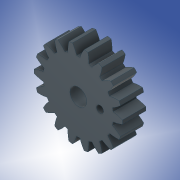
# Autodesk Inventor part: GA002
Saved by Autodesk Inventor 2017 SP1 (Build 210196100, 196)
## iProperties
Created: 2017-06-20
Part Number: GA002
Material: ABS Plastic
Document SubType Name: Modeling
Designer: zallen
Density: 1.06 g/cm^3
Appearance: CR Dark Blue
Author: zallen
Autodesk Inventor part; units mm, degrees
ref_plane "YZ Plane" through (0, 0, 0) normal (1, 0, 0) x (0, 1, 0)
ref_plane "XZ Plane" through (0, 0, 0) normal (0, 1, 0) x (-1, 0, 0)
ref_plane "XY Plane" through (0, 0, 0) normal (0, 0, 1) x (1, 0, 0)
sketch "Sketch1" plane through (0, 0, 0) normal (0, 0, 1) x (1, 0, 0)
  circle A0 centre (0, 0) radius 15
  circle A1 centre (0, 0) radius 3.6
  dimension "d0" = 30
  dimension "d1" = 7.2
  constraints: 2 centre point, 2 coincident
  measures "d0" diameter of A0
  measures "d1" diameter of A1
extrude "Extrusion1" add sketch "Sketch1" along normal blind 10
sketch "Sketch2" plane through (0, 0, 10) normal (0, 0, 1) x (1, 0, 0)
  circle A0 centre (9.3, 0) radius 1.5
  circle A1 centre (0, 0) radius 15 construction
  circle A2 centre (0, 0) radius 3.6 construction
  line L0 (3.6, 0) -> (15, 0) construction
  circle A3 centre (0, 0) radius 3.6 construction
  circle A4 centre (0, 0) radius 15 construction
  dimension "d4" = 3
  constraints: 5 horizontal alignment, 2 coincident, 2 end point, 1 centre point, 1 horizontal, 1 midpoint, 4 other
  measures "d4" diameter of A0
extrude "Extrusion2" cut sketch "Sketch2" against normal through all
sketch "Sketch3" plane through (0, 0, 10) normal (0, 0, 1) x (1, 0, 0)
  line L0 (0, 0) -> (25, 0) construction
  arc A0 (18.8792, 0.8) -> (14.8792, 1.9) centre (12.94, -12.9741) ccw
  circle A1 centre (0, 0) radius 15 projected
  arc A2 (18.8792, -0.8) -> (18.8792, 0.8) centre (-1.1048, 0) ccw
  arc A3 (14.8792, -1.9) -> (18.8792, -0.8) centre (12.94, 12.9741) ccw
  arc A4 (14.8792, -1.9) -> (14.8792, 1.9) centre (0, 0) ccw
  arc A5 (17.467, 7.2088) -> (13.332, 6.8744) centre (16.5971, -7.7659) ccw
  arc A6 (18.0142, 5.7053) -> (17.467, 7.2088) centre (-1.0382, -0.3779) ccw
  arc A7 (14.6317, 3.3036) -> (18.0142, 5.7053) centre (7.7223, 16.6175) ccw
  arc A8 (14.6317, 3.3036) -> (13.332, 6.8744) centre (0, 0) ccw
  arc A9 (13.9481, 12.7481) -> (10.1768, 11.0196) centre (18.2523, -1.6211) ccw
  arc A10 (14.9765, 11.5225) -> (13.9481, 12.7481) centre (-0.8463, -0.7102) ccw
  arc A11 (12.6194, 8.1087) -> (14.9765, 11.5225) centre (1.573, 18.2565) ccw
  arc A12 (12.6194, 8.1087) -> (10.1768, 11.0196) centre (0, 0) ccw
  arc A13 (8.7468, 16.7498) -> (5.7941, 13.8357) centre (17.7059, 4.7193) ccw
  arc A14 (10.1324, 15.9498) -> (8.7468, 16.7498) centre (-0.5524, -0.9568) ccw
  arc A15 (9.085, 11.9357) -> (10.1324, 15.9498) centre (-4.7659, 17.6935) ccw
  arc A16 (9.085, 11.9357) -> (5.7941, 13.8357) centre (0, 0) ccw
  arc A17 (2.4905, 18.7313) -> (0.7126, 14.9831) centre (15.024, 10.4905) ccw
  arc A18 (4.0662, 18.4534) -> (2.4905, 18.7313) centre (-0.1918, -1.088) ccw
  arc A19 (4.4549, 14.3232) -> (4.0662, 18.4534) centre (-10.53, 14.9964) ccw
  arc A20 (4.4549, 14.3232) -> (0.7126, 14.9831) centre (0, 0) ccw
  arc A21 (-4.0662, 18.4534) -> (-4.4549, 14.3232) centre (10.53, 14.9964) ccw
  arc A22 (-2.4905, 18.7313) -> (-4.0662, 18.4534) centre (0.1918, -1.088) ccw
  arc A23 (-0.7126, 14.9831) -> (-2.4905, 18.7313) centre (-15.024, 10.4905) ccw
  arc A24 (-0.7126, 14.9831) -> (-4.4549, 14.3232) centre (0, 0) ccw
  arc A25 (-10.1324, 15.9498) -> (-9.085, 11.9357) centre (4.7659, 17.6935) ccw
  arc A26 (-8.7468, 16.7498) -> (-10.1324, 15.9498) centre (0.5524, -0.9568) ccw
  arc A27 (-5.7941, 13.8357) -> (-8.7468, 16.7498) centre (-17.7059, 4.7193) ccw
  arc A28 (-5.7941, 13.8357) -> (-9.085, 11.9357) centre (0, 0) ccw
  arc A29 (-14.9765, 11.5225) -> (-12.6194, 8.1087) centre (-1.573, 18.2565) ccw
  arc A30 (-13.9481, 12.7481) -> (-14.9765, 11.5225) centre (0.8463, -0.7102) ccw
  arc A31 (-10.1768, 11.0196) -> (-13.9481, 12.7481) centre (-18.2523, -1.6211) ccw
  arc A32 (-10.1768, 11.0196) -> (-12.6194, 8.1087) centre (0, 0) ccw
  arc A33 (-18.0142, 5.7053) -> (-14.6317, 3.3036) centre (-7.7223, 16.6175) ccw
  arc A34 (-17.467, 7.2088) -> (-18.0142, 5.7053) centre (1.0382, -0.3779) ccw
  arc A35 (-13.332, 6.8744) -> (-17.467, 7.2088) centre (-16.5971, -7.7659) ccw
  arc A36 (-13.332, 6.8744) -> (-14.6317, 3.3036) centre (0, 0) ccw
  arc A37 (-18.8792, -0.8) -> (-14.8792, -1.9) centre (-12.94, 12.9741) ccw
  arc A38 (-18.8792, 0.8) -> (-18.8792, -0.8) centre (1.1048, 0) ccw
  arc A39 (-14.8792, 1.9) -> (-18.8792, 0.8) centre (-12.94, -12.9741) ccw
  arc A40 (-14.8792, 1.9) -> (-14.8792, -1.9) centre (0, 0) ccw
  arc A41 (-17.467, -7.2088) -> (-13.332, -6.8744) centre (-16.5971, 7.7659) ccw
  arc A42 (-18.0142, -5.7053) -> (-17.467, -7.2088) centre (1.0382, 0.3779) ccw
  arc A43 (-14.6317, -3.3036) -> (-18.0142, -5.7053) centre (-7.7223, -16.6175) ccw
  arc A44 (-14.6317, -3.3036) -> (-13.332, -6.8744) centre (0, 0) ccw
  arc A45 (-13.9481, -12.7481) -> (-10.1768, -11.0196) centre (-18.2523, 1.6211) ccw
  arc A46 (-14.9765, -11.5225) -> (-13.9481, -12.7481) centre (0.8463, 0.7102) ccw
  arc A47 (-12.6194, -8.1087) -> (-14.9765, -11.5225) centre (-1.573, -18.2565) ccw
  arc A48 (-12.6194, -8.1087) -> (-10.1768, -11.0196) centre (0, 0) ccw
  arc A49 (-8.7468, -16.7498) -> (-5.7941, -13.8357) centre (-17.7059, -4.7193) ccw
  arc A50 (-10.1324, -15.9498) -> (-8.7468, -16.7498) centre (0.5524, 0.9568) ccw
  arc A51 (-9.085, -11.9357) -> (-10.1324, -15.9498) centre (4.7659, -17.6935) ccw
  arc A52 (-9.085, -11.9357) -> (-5.7941, -13.8357) centre (0, 0) ccw
  arc A53 (-2.4905, -18.7313) -> (-0.7126, -14.9831) centre (-15.024, -10.4905) ccw
  arc A54 (-4.0662, -18.4534) -> (-2.4905, -18.7313) centre (0.1918, 1.088) ccw
  arc A55 (-4.4549, -14.3232) -> (-4.0662, -18.4534) centre (10.53, -14.9964) ccw
  arc A56 (-4.4549, -14.3232) -> (-0.7126, -14.9831) centre (0, 0) ccw
  arc A57 (4.0662, -18.4534) -> (4.4549, -14.3232) centre (-10.53, -14.9964) ccw
  arc A58 (2.4905, -18.7313) -> (4.0662, -18.4534) centre (-0.1918, 1.088) ccw
  arc A59 (0.7126, -14.9831) -> (2.4905, -18.7313) centre (15.024, -10.4905) ccw
  arc A60 (0.7126, -14.9831) -> (4.4549, -14.3232) centre (0, 0) ccw
  arc A61 (10.1324, -15.9498) -> (9.085, -11.9357) centre (-4.7659, -17.6935) ccw
  arc A62 (8.7468, -16.7498) -> (10.1324, -15.9498) centre (-0.5524, 0.9568) ccw
  arc A63 (5.7941, -13.8357) -> (8.7468, -16.7498) centre (17.7059, -4.7193) ccw
  arc A64 (5.7941, -13.8357) -> (9.085, -11.9357) centre (0, 0) ccw
  arc A65 (14.9765, -11.5225) -> (12.6194, -8.1087) centre (1.573, -18.2565) ccw
  arc A66 (13.9481, -12.7481) -> (14.9765, -11.5225) centre (-0.8463, 0.7102) ccw
  arc A67 (10.1768, -11.0196) -> (13.9481, -12.7481) centre (18.2523, 1.6211) ccw
  arc A68 (10.1768, -11.0196) -> (12.6194, -8.1087) centre (0, 0) ccw
  arc A69 (18.0142, -5.7053) -> (14.6317, -3.3036) centre (7.7223, -16.6175) ccw
  arc A70 (17.467, -7.2088) -> (18.0142, -5.7053) centre (-1.0382, 0.3779) ccw
  arc A71 (13.332, -6.8744) -> (17.467, -7.2088) centre (16.5971, 7.7659) ccw
  arc A72 (13.332, -6.8744) -> (14.6317, -3.3036) centre (0, 0) ccw
  point P0 (18.8952, 0)
  point P1 (17.7557, 6.4625)
  point P2 (14.4746, 12.1456)
  point P3 (9.4476, 16.3637)
  point P4 (3.2811, 18.6081)
  point P5 (-3.2811, 18.6081)
  point P6 (-9.4476, 16.3637)
  point P7 (-14.4746, 12.1456)
  point P8 (-17.7557, 6.4625)
  point P9 (-18.8952, 0)
  point P10 (-17.7557, -6.4625)
  point P11 (-14.4746, -12.1456)
  point P12 (-9.4476, -16.3637)
  point P13 (-3.2811, -18.6081)
  point P14 (3.2811, -18.6081)
  point P15 (9.4476, -16.3637)
  point P16 (14.4746, -12.1456)
  point P17 (17.7557, -6.4625)
  dimension "d8" = 25
  dimension "d9" = 15
  dimension "d10" = 1.6
  dimension "d11" = 20
  dimension "d12" = 4
  dimension "d13" = 1.1
  dimension "d14" = 15
  dimension "d15" = 1.1
  dimension "d16" = 4
  dimension "d19" = 360
  constraints: 147 point on circle, 72 centre point, 2 end point, 1 concentric, 1 horizontal, 1 point on line, 235 other
  measures "d8" distance of L0.start L0.end
  measures "d9" radius of A0
  measures "d10" distance of A0.start A2.start
  measures "d11" radius of A2
  measures "d12" horizontal distance of A0.start A0.end
  measures "d13" vertical distance of A0.start A0.end
  measures "d14" radius of A3
  measures "d15" vertical distance of A2.start A1.end
  measures "d16" horizontal distance of A1.end A2.start
extrude "Extrusion3" add sketch "Sketch3" against normal blind 10 contours A2 A3 A1 A0 | A1 A5 A6 A7 | A69 A70 A71 A1 | A1 A9 A10 A11 | A65 A66 A67 A1 | A1 A13 A14 A15 | A61 A62 A63 A1 | A1 A17 A18 A19 | A57 A58 A59 A1 | A1 A21 A22 A23 | A53 A54 A55 A1 | A1 A25 A26 A27 | A49 A50 A51 A1 | A1 A29 A30 A31 | A45 A46 A47 A1 | A1 A33 A34 A35 | A41 A42 A43 A1 | A1 A37 A38 A39
body "Solid1"
